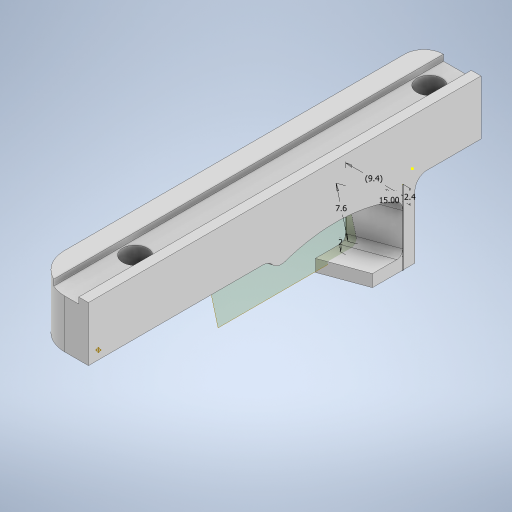
# Autodesk Inventor part: Right-Brush-Bottom
Saved by Autodesk Inventor 2024 (Build 280153000, 153)
## iProperties
Created: 2023-12-12
Part Number: Right-Brush-Bottom
Material: Generic
Document SubType Name: Modeling
Designer: shaun
Density: 1 g/cm^3
Appearance: Default
Author: shaun
Autodesk Inventor part; units mm, degrees
ref_plane "YZ Plane" through (0, 0, 0) normal (1, 0, 0) x (0, 1, 0)
ref_plane "XZ Plane" through (0, 0, 0) normal (0, 1, 0) x (-1, 0, 0)
ref_plane "XY Plane" through (0, 0, 0) normal (0, 0, 1) x (1, 0, 0)
sketch "Sketch1" plane through (0, 0, 0) normal (0, 1, 0) x (-1, 0, 0)
  line L0 (0, 0) -> (11, 0) construction
  line L1 (11, 0) -> (11, -64.7) construction
  line L2 (11, -64.7) -> (0, -64.7) construction
  line L3 (0, -64.7) -> (0, 0) construction
  line L4 (5.5, 0) -> (5.5, -64.7) construction
  line L5 (11, -32.35) -> (0, -32.35) construction
  circle A0 centre (5.5, -11.6) radius 1.6 construction
  circle A1 centre (5.5, -11.6) radius 2.05
  circle A2 centre (5.5, -21.3) radius 1.6 construction
  circle A3 centre (5.5, -21.3) radius 2.05 construction
  circle A4 centre (5.5, -31) radius 1.6 construction
  circle A5 centre (5.5, -31) radius 2.05 construction
  circle A6 centre (5.5, -40.7) radius 1.6 construction
  circle A7 centre (5.5, -40.7) radius 2.05 construction
  circle A8 centre (5.5, -50.4) radius 1.6 construction
  circle A9 centre (5.5, -50.4) radius 2.05 construction
  circle A10 centre (5.5, -60.1) radius 1.6 construction
  circle A11 centre (5.5, -60.1) radius 2.05
  line L6 (7.8, 0) -> (3.2, 0) construction
  line L7 (3.2, 0) -> (3.2, -64.7)
  line L8 (3.2, -64.7) -> (7.8, -64.7) construction
  line L9 (7.8, -64.7) -> (7.8, 0)
  circle A12 centre (5.5, -11.6) radius 2.3 construction
  circle A13 centre (5.5, -5.5) radius 5.5 construction
  circle A14 centre (7.8, -61.5) radius 3.2 construction
  line L10 (0, -64.7) -> (3.2, -64.7) construction
  line L11 (1.6, -64.7) -> (1.6, 0)
  circle A15 centre (5.5, -60.1) radius 3.5
  circle A16 centre (5.5, -50.4) radius 3.5 construction
  circle A17 centre (5.5, -40.7) radius 3.5 construction
  circle A18 centre (5.5, -31) radius 3.5 construction
  circle A19 centre (5.5, -21.3) radius 3.5 construction
  circle A20 centre (5.5, -11.6) radius 3.5
  arc A21 (7.8, -64.7) -> (11, -61.5) centre (7.8, -61.5) ccw
  arc A22 (11, -5.5) -> (5.5, 0) centre (5.5, -5.5) ccw
  line L12 (11, -61.5) -> (11, -5.5)
  line L13 (1.6, -64.7) -> (7.8, -64.7)
  line L14 (1.6, 0) -> (5.5, 0)
  point P0 (5.5, -10)
  point P1 (5.5, -61.7)
  point P2 (7.8, -0.504)
  dimension "d0" = 3.2
  dimension "d1" = 4.1
  dimension "d4" = 9.7
  dimension "d9" = 6.5
  dimension "d10" = 10
  dimension "d11" = 3
  dimension "d12" = 0.7
  dimension "d13" = 3.2
  dimension "d14" = 7
  constraints: 30 end point, 21 centre point, 16 coincident, 10 point on line, 8 point on circle, 5 equal radius, 5 midpoint, 5 parallel, 5 tangent, 3 perpendicular, 2 collinear, 2 horizontal, 2 line through centre, 2 vertical, 2 vertical alignment, 22 other
  measures "d1" diameter of A1
  measures "d4" distance of point (5.5, -11.6) A2.centre
  measures "d10" distance from line of L0 point (5.5, -10)
  measures "d11" distance of L4.end point (5.5, -61.7)
  measures "d13" distance between parallel lines of L1 L9
  measures "d14" diameter of A15
extrude "Extrusion1" add sketch "Sketch1" along normal blind 6 contours L7 A20 A15 L13 L11 L14 | L7 A20 | A20 L9 | L9 A22 L12 A21 A15 A20 | L7 A15 | A15 L9
extrude "Extrusion3" add sketch "Sketch1" along normal blind 5 contours L14 A22 L9 A20 L7 | A20 L9 L7 | A20 L9 A15 L7 | A15 L9 L7 | L7 A15 L9 L13
extrude "Extrusion2" add sketch "Sketch1" against normal blind 3 contours L14 A22 L9 A20 L7 | L7 A20 A15 L13 L11 L14 | A20 L9 A15 L7 | L9 A22 L12 A21 A15 A20 | L7 A15 L9 L13
sketch "Sketch2" plane through (0, -3, 0) normal (0, -1, 0) x (1, 0, 0)
  line L0 (-1.6, -64.7) -> (-1.6, 0) construction
  circle A0 centre (-5.5, -11.6) radius 3.5 construction
  circle A1 centre (-5.5, -60.1) radius 3.5 construction
  line L1 (-11, -5.5) -> (-11, -61.5) construction
  arc A2 (-11, -61.5) -> (-7.8, -64.7) centre (-7.8, -61.5) ccw construction
  line L2 (-7.8, -64.7) -> (-1.6, -64.7) construction
  arc A3 (-5.5, 0) -> (-11, -5.5) centre (-5.5, -5.5) ccw construction
  line L3 (-1.6, 0) -> (-5.5, 0) construction
  line L4 (-5.5, -60.1) -> (-5.5, -11.6) construction
  circle A4 centre (-5.5, -55.25) radius 4.85 construction
  circle A5 centre (-5.5, -45.55) radius 4.85 construction
  circle A6 centre (-5.5, -35.85) radius 4.85 construction
  circle A7 centre (-5.5, -26.15) radius 4.85 construction
  circle A8 centre (-5.5, -16.45) radius 4.85 construction
  line L5 (0, -51.8) -> (-11, -51.8) construction
  line L6 (-11, -51.8) -> (-11, -29.6) construction
  line L7 (-11, -29.6) -> (0, -29.6) construction
  line L8 (0, -29.6) -> (0, -51.8) construction
  line L9 (0, -51.8) -> (-11, -29.6) construction
  line L10 (-11, -51.8) -> (0, -29.6) construction
  line L11 (0, -27.1) -> (-11, -27.1) construction
  line L12 (-11, -27.1) -> (-11, -54.3) construction
  line L13 (-11, -54.3) -> (0, -54.3) construction
  line L14 (0, -54.3) -> (0, -27.1) construction
  line L15 (0, -27.1) -> (-11, -54.3) construction
  line L16 (-11, -27.1) -> (0, -54.3) construction
  line L17 (-11, -54.3) -> (-1.6, -54.3)
  line L18 (-1.6, -54.3) -> (-1.6, -51.8)
  line L19 (-1.6, -51.8) -> (-11, -51.8)
  line L20 (-11, -51.8) -> (-11, -54.3)
  point P0 (0, 0)
  point P1 (-5.5, -50.4)
  point P2 (-5.5, -40.7)
  point P3 (-5.5, -31)
  point P4 (-5.5, -21.3)
  dimension "d21" = 22.2
  dimension "d22" = 2.5
  constraints: 32 end point, 10 point on circle, 6 parallel, 5 centre point, 4 equal radius, 4 midpoint, 4 point on line, 3 horizontal, 3 perpendicular, 12 other
  measures "d21" distance of L5.end L6.end
  measures "d22" distance between parallel lines of L5 L13
ref_plane "Work Plane1" through (-1.6, -3, -51.8) normal (0, 0, 1) x (1, 0, 0)
sketch "Sketch3" plane through (-1.6, -3, -51.8) normal (0, 0, 1) x (1, 0, 0)
  line L0 (0, 0) -> (-9.4, 0) projected
  line L1 (0, 0) -> (0, -2.4)
  line L2 (0, -2.4) -> (-9.4, -4.9187)
  line L3 (-9.4, -4.9187) -> (-9.4, 0)
  line L4 (0, -2.4) -> (-9.4, -2.4) construction
  line L5 (0, -2.4) -> (0, -10.2681)
  line L6 (0, -10.2681) -> (-9.4, -12.7868)
  line L7 (-9.4, -12.7868) -> (-9.4, -4.9187)
  line L8 (-9.4, -12.7868) -> (-9.4, -14.7868)
  line L9 (-9.4, -14.7868) -> (0, -12.2681)
  line L10 (0, -12.2681) -> (0, -10.2681)
  line L11 (-9.4, -4.9187) -> (-7.433, -12.2598) construction
  point P0 (1.6, 3)
  dimension "d23" = 2.4
  dimension "d24" = 15
  dimension "d25" = 9.4
  dimension "d26" = 2
  dimension "d27" = 7.6
  constraints: 22 end point, 4 parallel, 4 point on line, 3 perpendicular, 2 vertical
  measures "d23" distance of L0.start L1.end
  measures "d24" angle of L4 L2
  measures "d25" distance of L1.end L4.end
  measures "d26" distance of L8.end L6.end
  measures "d27" distance of L2.end L11.end
extrude "Extrusion4" add sketch "Sketch3" against normal blind 2
extrude "Extrusion5" add sketch "Sketch3" along normal blind 22 contours L1 L2 L3 L0
ref_plane "Work Plane2" through (-11, -7.9187, -51.8) normal (-0.9659258, -0.258819, 0) x (0.258819, -0.9659258, 0)
sketch "Sketch4" plane through (-11, -7.9187, -51.8) normal (-0.9659258, -0.258819, 0) x (0.258819, -0.9659258, 0)
  line L0 (0, 0) -> (0, 22) projected
  arc A0 (0, 22) -> (0, 0) centre (24.0083, 11) ccw
  point P0 (-4.8019, 51.8)
  point P1 (-2.4, 11)
  point P2 (0, 11)
  dimension "d32" = 2.4
  constraints: 3 point on circle, 1 centre point, 1 midpoint
  measures "d32" distance of point (-2.4, 11) point (0, 11)
extrude "Extrusion6" cut sketch "Sketch4" against normal through all
extrude "Extrusion7" add sketch "Sketch3" along normal blind 5 contours L10 L9 L8 L6
fillet "Fillet1" radius 2 4 edges at (-6.3, -6.6594, -29.8) (-6.3, -3, -29.8) (-6.3, -3, -53.8) (-6.3, -6.6594, -51.8)
fillet "Fillet2" radius 1 1 edges at (-6.3, -14.5275, -51.8)
body "Solid1"
